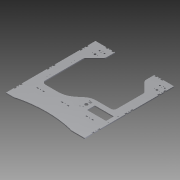
# Autodesk Inventor part: pieza frontal nueva
Saved by Autodesk Inventor 2012 SP1 (Build 160190100, 190)
## iProperties
Created: 2014-12-15
Part Number: pieza frontal nueva
Material: Default
Document SubType Name: Modeling
Designer: PRINCIPAL
Density: 1 g/cm^3
Author: PRINCIPAL
Autodesk Inventor part; units mm, degrees
ref_plane "YZ Plane" through (0, 0, 0) normal (1, 0, 0) x (0, 1, 0)
ref_plane "XZ Plane" through (0, 0, 0) normal (0, 1, 0) x (-1, 0, 0)
ref_plane "XY Plane" through (0, 0, 0) normal (0, 0, 1) x (1, 0, 0)
sketch "Boceto1" plane through (0, 0, 0) normal (0, 0, 1) x (1, 0, 0)
  arc A0 (-182.0823, -56.4965) -> (-184.1823, -54.3965) centre (-184.1823, -56.4965) ccw
  arc A1 (-184.1823, -58.5965) -> (-182.0823, -56.4965) centre (-184.1823, -56.4965) ccw
  arc A2 (-186.2823, -56.4965) -> (-184.1823, -58.5965) centre (-184.1823, -56.4965) ccw
  arc A3 (-184.1823, -54.3965) -> (-186.2823, -56.4965) centre (-184.1823, -56.4965) ccw
  arc A4 (212.9177, -56.4965) -> (210.8177, -54.3965) centre (210.8177, -56.4965) ccw
  arc A5 (210.8177, -58.5965) -> (212.9177, -56.4965) centre (210.8177, -56.4965) ccw
  arc A6 (208.7177, -56.4965) -> (210.8177, -58.5965) centre (210.8177, -56.4965) ccw
  arc A7 (210.8177, -54.3965) -> (208.7177, -56.4965) centre (210.8177, -56.4965) ccw
  arc A8 (206.3177, -154.7797) -> (204.3177, -152.7797) centre (204.3177, -154.7797) ccw
  arc A9 (204.3177, -156.7797) -> (206.3177, -154.7797) centre (204.3177, -154.7797) ccw
  arc A10 (202.3177, -154.7797) -> (204.3177, -156.7797) centre (204.3177, -154.7797) ccw
  arc A11 (204.3177, -152.7797) -> (202.3177, -154.7797) centre (204.3177, -154.7797) ccw
  arc A12 (62.3177, -104.7797) -> (60.3177, -102.7797) centre (60.3177, -104.7797) ccw
  arc A13 (60.3177, -106.7797) -> (62.3177, -104.7797) centre (60.3177, -104.7797) ccw
  arc A14 (58.3177, -104.7797) -> (60.3177, -106.7797) centre (60.3177, -104.7797) ccw
  arc A15 (60.3177, -102.7797) -> (58.3177, -104.7797) centre (60.3177, -104.7797) ccw
  arc A16 (62.3177, -154.7797) -> (60.3177, -152.7797) centre (60.3177, -154.7797) ccw
  arc A17 (60.3177, -156.7797) -> (62.3177, -154.7797) centre (60.3177, -154.7797) ccw
  arc A18 (58.3177, -154.7797) -> (60.3177, -156.7797) centre (60.3177, -154.7797) ccw
  arc A19 (60.3177, -152.7797) -> (58.3177, -154.7797) centre (60.3177, -154.7797) ccw
  arc A20 (206.3177, -104.7797) -> (204.3177, -102.7797) centre (204.3177, -104.7797) ccw
  arc A21 (204.3177, -106.7797) -> (206.3177, -104.7797) centre (204.3177, -104.7797) ccw
  arc A22 (202.3177, -104.7797) -> (204.3177, -106.7797) centre (204.3177, -104.7797) ccw
  arc A23 (204.3177, -102.7797) -> (202.3177, -104.7797) centre (204.3177, -104.7797) ccw
  line L0 (148.3677, -185.9715) -> (158.2677, -185.9715)
  line L1 (158.2677, -185.9715) -> (158.2677, -181.0215)
  line L2 (158.2677, -181.0215) -> (148.3677, -181.0215)
  line L3 (148.3677, -181.0215) -> (148.3677, -185.9715)
  line L4 (33.2677, -185.9715) -> (33.2677, -181.0215)
  line L5 (33.2677, -181.0215) -> (23.3677, -181.0215)
  line L6 (23.3677, -181.0215) -> (23.3677, -185.9715)
  line L7 (23.3677, -185.9715) -> (33.2677, -185.9715)
  line L8 (-91.7323, -185.9715) -> (-91.7323, -181.0215)
  line L9 (-91.7323, -181.0215) -> (-101.6323, -181.0215)
  line L10 (-101.6323, -181.0215) -> (-101.6323, -185.9715)
  line L11 (-101.6323, -185.9715) -> (-91.7323, -185.9715)
  line L12 (3.2677, -185.9715) -> (3.2677, -181.0215)
  line L13 (3.2677, -181.0215) -> (-6.6323, -181.0215)
  line L14 (-6.6323, -181.0215) -> (-6.6323, -185.9715)
  line L15 (-6.6323, -185.9715) -> (3.2677, -185.9715)
  line L16 (-121.7323, -185.9715) -> (-121.7323, -181.0215)
  line L17 (-121.7323, -181.0215) -> (-131.6323, -181.0215)
  line L18 (-131.6323, -181.0215) -> (-131.6323, -185.9715)
  line L19 (-131.6323, -185.9715) -> (-121.7323, -185.9715)
  arc A24 (-109.6823, -183.4965) -> (-111.6823, -181.4965) centre (-111.6823, -183.4965) ccw
  arc A25 (-111.6823, -185.4965) -> (-109.6823, -183.4965) centre (-111.6823, -183.4965) ccw
  arc A26 (-113.6823, -183.4965) -> (-111.6823, -185.4965) centre (-111.6823, -183.4965) ccw
  arc A27 (-111.6823, -181.4965) -> (-113.6823, -183.4965) centre (-111.6823, -183.4965) ccw
  arc A28 (-182.1823, -224.4965) -> (-184.1823, -222.4965) centre (-184.1823, -224.4965) ccw
  arc A29 (-184.1823, -226.4965) -> (-182.1823, -224.4965) centre (-184.1823, -224.4965) ccw
  arc A30 (-186.1823, -224.4965) -> (-184.1823, -226.4965) centre (-184.1823, -224.4965) ccw
  arc A31 (-184.1823, -222.4965) -> (-186.1823, -224.4965) centre (-184.1823, -224.4965) ccw
  arc A32 (15.3177, -183.4965) -> (13.3177, -181.4965) centre (13.3177, -183.4965) ccw
  arc A33 (13.3177, -185.4965) -> (15.3177, -183.4965) centre (13.3177, -183.4965) ccw
  arc A34 (11.3177, -183.4965) -> (13.3177, -185.4965) centre (13.3177, -183.4965) ccw
  arc A35 (13.3177, -181.4965) -> (11.3177, -183.4965) centre (13.3177, -183.4965) ccw
  arc A36 (140.3177, -183.4965) -> (138.3177, -181.4965) centre (138.3177, -183.4965) ccw
  arc A37 (138.3177, -185.4965) -> (140.3177, -183.4965) centre (138.3177, -183.4965) ccw
  arc A38 (136.3177, -183.4965) -> (138.3177, -185.4965) centre (138.3177, -183.4965) ccw
  arc A39 (138.3177, -181.4965) -> (136.3177, -183.4965) centre (138.3177, -183.4965) ccw
  arc A40 (212.8177, -224.4965) -> (210.8177, -222.4965) centre (210.8177, -224.4965) ccw
  arc A41 (210.8177, -226.4965) -> (212.8177, -224.4965) centre (210.8177, -224.4965) ccw
  arc A42 (208.8177, -224.4965) -> (210.8177, -226.4965) centre (210.8177, -224.4965) ccw
  arc A43 (210.8177, -222.4965) -> (208.8177, -224.4965) centre (210.8177, -224.4965) ccw
  line L20 (118.3677, -185.9715) -> (128.2677, -185.9715)
  line L21 (128.2677, -185.9715) -> (128.2677, -181.0215)
  line L22 (128.2677, -181.0215) -> (118.3677, -181.0215)
  line L23 (118.3677, -181.0215) -> (118.3677, -185.9715)
  line L24 (64.9824, -107.508) -> (64.9824, -109.0513)
  line L25 (64.9824, -109.0513) -> (77.3177, -109.0513)
  line L26 (77.3177, -109.0513) -> (77.3177, -107.508)
  line L27 (77.3177, -107.508) -> (64.9824, -107.508)
  line L28 (64.9824, -116.5513) -> (64.9824, -118.0513)
  line L29 (64.9824, -118.0513) -> (77.3177, -118.0513)
  line L30 (77.3177, -118.0513) -> (77.3177, -116.5513)
  line L31 (77.3177, -116.5513) -> (64.9824, -116.5513)
  line L32 (64.9824, -113.5513) -> (64.9824, -115.0513)
  line L33 (64.9824, -115.0513) -> (77.3177, -115.0513)
  line L34 (77.3177, -115.0513) -> (77.3177, -113.5513)
  line L35 (77.3177, -113.5513) -> (64.9824, -113.5513)
  line L36 (77.3177, -112.0513) -> (77.3177, -110.5513)
  line L37 (77.3177, -110.5513) -> (64.9824, -110.5513)
  line L38 (64.9824, -110.5513) -> (64.9824, -112.0513)
  line L39 (64.9824, -112.0513) -> (77.3177, -112.0513)
  arc A44 (72.3677, -148.9787) -> (70.3177, -146.9287) centre (70.3177, -148.9787) ccw
  arc A45 (70.3177, -151.0287) -> (72.3677, -148.9787) centre (70.3177, -148.9787) ccw
  arc A46 (68.2677, -148.9787) -> (70.3177, -151.0287) centre (70.3177, -148.9787) ccw
  arc A47 (70.3177, -146.9287) -> (68.2677, -148.9787) centre (70.3177, -148.9787) ccw
  line L40 (193.1177, -115.2675) -> (193.1177, -154.2918)
  arc A48 (192.8475, -154.5619) -> (193.1177, -154.2918) centre (192.8475, -154.2918) ccw
  line L41 (192.8475, -154.5619) -> (96.7879, -154.5619)
  arc A49 (96.5177, -154.2918) -> (96.7879, -154.5619) centre (96.7879, -154.2918) ccw
  line L42 (96.5177, -154.2918) -> (96.5177, -115.2675)
  arc A50 (96.7879, -114.9974) -> (96.5177, -115.2675) centre (96.7879, -115.2675) ccw
  line L43 (96.7879, -114.9974) -> (192.8475, -114.9974)
  arc A51 (193.1177, -115.2675) -> (192.8475, -114.9974) centre (192.8475, -115.2675) ccw
  arc A52 (62.3177, -132.2797) -> (70.3177, -140.2797) centre (70.3177, -132.2797) ccw
  arc A53 (70.3177, -124.2797) -> (62.3177, -132.2797) centre (70.3177, -132.2797) ccw
  arc A54 (78.3177, -132.2797) -> (70.3177, -124.2797) centre (70.3177, -132.2797) ccw
  arc A55 (70.3177, -140.2797) -> (78.3177, -132.2797) centre (70.3177, -132.2797) ccw
  arc A56 (173.8177, 142.5277) -> (170.3177, 139.0277) centre (173.8177, 139.0277) ccw
  arc A57 (170.3177, 139.0277) -> (173.8177, 135.5277) centre (173.8177, 139.0277) ccw
  arc A58 (173.8177, 135.5277) -> (177.3177, 139.0277) centre (173.8177, 139.0277) ccw
  arc A59 (177.3177, 139.0277) -> (173.8177, 142.5277) centre (173.8177, 139.0277) ccw
  arc A60 (198.8177, 142.5277) -> (195.3177, 139.0277) centre (198.8177, 139.0277) ccw
  arc A61 (195.3177, 139.0277) -> (198.8177, 135.5277) centre (198.8177, 139.0277) ccw
  arc A62 (198.8177, 135.5277) -> (202.3177, 139.0277) centre (198.8177, 139.0277) ccw
  arc A63 (202.3177, 139.0277) -> (198.8177, 142.5277) centre (198.8177, 139.0277) ccw
  arc A64 (186.3177, 135.5777) -> (184.7677, 134.0277) centre (186.3177, 134.0277) ccw
  arc A65 (184.7677, 134.0277) -> (186.3177, 132.4777) centre (186.3177, 134.0277) ccw
  arc A66 (186.3177, 132.4777) -> (187.8677, 134.0277) centre (186.3177, 134.0277) ccw
  arc A67 (187.8677, 134.0277) -> (186.3177, 135.5777) centre (186.3177, 134.0277) ccw
  arc A68 (186.3177, 145.5777) -> (184.7677, 144.0277) centre (186.3177, 144.0277) ccw
  arc A69 (184.7677, 144.0277) -> (186.3177, 142.4777) centre (186.3177, 144.0277) ccw
  arc A70 (186.3177, 142.4777) -> (187.8677, 144.0277) centre (186.3177, 144.0277) ccw
  arc A71 (187.8677, 144.0277) -> (186.3177, 145.5777) centre (186.3177, 144.0277) ccw
  arc A72 (-108.1823, 142.5277) -> (-111.6823, 139.0277) centre (-108.1823, 139.0277) ccw
  arc A73 (-111.6823, 139.0277) -> (-108.1823, 135.5277) centre (-108.1823, 139.0277) ccw
  arc A74 (-108.1823, 135.5277) -> (-104.6823, 139.0277) centre (-108.1823, 139.0277) ccw
  arc A75 (-104.6823, 139.0277) -> (-108.1823, 142.5277) centre (-108.1823, 139.0277) ccw
  arc A76 (-133.1823, 142.5277) -> (-136.6823, 139.0277) centre (-133.1823, 139.0277) ccw
  arc A77 (-136.6823, 139.0277) -> (-133.1823, 135.5277) centre (-133.1823, 139.0277) ccw
  arc A78 (-133.1823, 135.5277) -> (-129.6823, 139.0277) centre (-133.1823, 139.0277) ccw
  arc A79 (-129.6823, 139.0277) -> (-133.1823, 142.5277) centre (-133.1823, 139.0277) ccw
  arc A80 (-120.6823, 135.5777) -> (-122.2323, 134.0277) centre (-120.6823, 134.0277) ccw
  arc A81 (-122.2323, 134.0277) -> (-120.6823, 132.4777) centre (-120.6823, 134.0277) ccw
  arc A82 (-120.6823, 132.4777) -> (-119.1323, 134.0277) centre (-120.6823, 134.0277) ccw
  arc A83 (-119.1323, 134.0277) -> (-120.6823, 135.5777) centre (-120.6823, 134.0277) ccw
  arc A84 (-120.6823, 145.5777) -> (-122.2323, 144.0277) centre (-120.6823, 144.0277) ccw
  arc A85 (-122.2323, 144.0277) -> (-120.6823, 142.4777) centre (-120.6823, 144.0277) ccw
  arc A86 (-120.6823, 142.4777) -> (-119.1323, 144.0277) centre (-120.6823, 144.0277) ccw
  arc A87 (-119.1323, 144.0277) -> (-120.6823, 145.5777) centre (-120.6823, 144.0277) ccw
  arc A88 (173.8177, 113.0777) -> (172.2677, 111.5277) centre (173.8177, 111.5277) ccw
  arc A89 (172.2677, 111.5277) -> (173.8177, 109.9777) centre (173.8177, 111.5277) ccw
  arc A90 (173.8177, 109.9777) -> (175.3677, 111.5277) centre (173.8177, 111.5277) ccw
  arc A91 (175.3677, 111.5277) -> (173.8177, 113.0777) centre (173.8177, 111.5277) ccw
  arc A92 (-116.6823, 113.0777) -> (-118.2323, 111.5277) centre (-116.6823, 111.5277) ccw
  arc A93 (-118.2323, 111.5277) -> (-116.6823, 109.9777) centre (-116.6823, 111.5277) ccw
  arc A94 (-116.6823, 109.9777) -> (-115.1323, 111.5277) centre (-116.6823, 111.5277) ccw
  arc A95 (-115.1323, 111.5277) -> (-116.6823, 113.0777) centre (-116.6823, 111.5277) ccw
  arc A96 (-141.6823, 113.0777) -> (-143.2323, 111.5277) centre (-141.6823, 111.5277) ccw
  arc A97 (-143.2323, 111.5277) -> (-141.6823, 109.9777) centre (-141.6823, 111.5277) ccw
  arc A98 (-141.6823, 109.9777) -> (-140.1323, 111.5277) centre (-141.6823, 111.5277) ccw
  arc A99 (-140.1323, 111.5277) -> (-141.6823, 113.0777) centre (-141.6823, 111.5277) ccw
  arc A100 (198.8177, 113.0777) -> (197.2677, 111.5277) centre (198.8177, 111.5277) ccw
  arc A101 (197.2677, 111.5277) -> (198.8177, 109.9777) centre (198.8177, 111.5277) ccw
  arc A102 (198.8177, 109.9777) -> (200.3677, 111.5277) centre (198.8177, 111.5277) ccw
  arc A103 (200.3677, 111.5277) -> (198.8177, 113.0777) centre (198.8177, 111.5277) ccw
  arc A104 (-111.6823, 171.0277) -> (-113.6823, 169.0277) centre (-111.6823, 169.0277) ccw
  arc A105 (-113.6823, 169.0277) -> (-111.6823, 167.0277) centre (-111.6823, 169.0277) ccw
  arc A106 (-111.6823, 167.0277) -> (-109.6823, 169.0277) centre (-111.6823, 169.0277) ccw
  arc A107 (-109.6823, 169.0277) -> (-111.6823, 171.0277) centre (-111.6823, 169.0277) ccw
  arc A108 (-184.1823, 113.5277) -> (-186.1823, 111.5277) centre (-184.1823, 111.5277) ccw
  arc A109 (-186.1823, 111.5277) -> (-184.1823, 109.5277) centre (-184.1823, 111.5277) ccw
  arc A110 (-184.1823, 109.5277) -> (-182.1823, 111.5277) centre (-184.1823, 111.5277) ccw
  arc A111 (-182.1823, 111.5277) -> (-184.1823, 113.5277) centre (-184.1823, 111.5277) ccw
  arc A112 (210.8177, 113.5277) -> (208.8177, 111.5277) centre (210.8177, 111.5277) ccw
  arc A113 (208.8177, 111.5277) -> (210.8177, 109.5277) centre (210.8177, 111.5277) ccw
  arc A114 (210.8177, 109.5277) -> (212.8177, 111.5277) centre (210.8177, 111.5277) ccw
  arc A115 (212.8177, 111.5277) -> (210.8177, 113.5277) centre (210.8177, 111.5277) ccw
  arc A116 (138.3177, 171.0277) -> (136.3177, 169.0277) centre (138.3177, 169.0277) ccw
  arc A117 (136.3177, 169.0277) -> (138.3177, 167.0277) centre (138.3177, 169.0277) ccw
  arc A118 (138.3177, 167.0277) -> (140.3177, 169.0277) centre (138.3177, 169.0277) ccw
  arc A119 (140.3177, 169.0277) -> (138.3177, 171.0277) centre (138.3177, 169.0277) ccw
  arc A120 (-129.1823, 116.7277) -> (-134.3823, 111.5277) centre (-129.1823, 111.5277) ccw
  arc A121 (-134.3823, 111.5277) -> (-129.1823, 106.3277) centre (-129.1823, 111.5277) ccw
  arc A122 (-129.1823, 106.3277) -> (-123.9823, 111.5277) centre (-129.1823, 111.5277) ccw
  arc A123 (-123.9823, 111.5277) -> (-129.1823, 116.7277) centre (-129.1823, 111.5277) ccw
  arc A124 (186.3177, 116.7277) -> (181.1177, 111.5277) centre (186.3177, 111.5277) ccw
  arc A125 (181.1177, 111.5277) -> (186.3177, 106.3277) centre (186.3177, 111.5277) ccw
  arc A126 (186.3177, 106.3277) -> (191.5177, 111.5277) centre (186.3177, 111.5277) ccw
  arc A127 (191.5177, 111.5277) -> (186.3177, 116.7277) centre (186.3177, 111.5277) ccw
  line L44 (-92.4695, 115.209) -> (-136.2182, 71.4603)
  arc A128 (-136.2182, 71.4603) -> (-140.5823, 60.9244) centre (-125.6823, 60.9244) ccw
  line L45 (-140.5823, 60.9244) -> (-140.5823, -129.0297)
  arc A129 (-140.5823, -129.0297) -> (-120.6823, -148.9297) centre (-120.6823, -129.0297) ccw
  line L46 (-120.6823, -148.9297) -> (-56.306, -148.9297)
  arc A130 (-56.306, -148.9297) -> (0.3907, -131.2823) centre (-56.306, -49.0297) ccw
  arc A131 (0.3907, -131.2823) -> (28.9935, -108.1231) centre (-135.1799, 65.3964) ccw
  arc A132 (77.1714, -88.9436) -> (28.9935, -108.1231) centre (77.1714, -159.0436) ccw
  line L47 (77.1714, -88.9436) -> (152.2606, -88.9436)
  arc A133 (152.2606, -88.9436) -> (167.1606, -74.0436) centre (152.2606, -74.0436) ccw
  line L48 (167.1606, -74.0436) -> (167.1606, 60.9244)
  arc A134 (167.1606, 60.9244) -> (162.7965, 71.4603) centre (152.2606, 60.9244) ccw
  line L49 (162.7965, 71.4603) -> (119.1048, 115.152)
  arc A135 (113.2177, 129.3648) -> (119.1048, 115.152) centre (133.3177, 129.3648) ccw
  line L50 (113.2177, 129.3648) -> (113.2177, 171.6035)
  line L51 (113.2177, 171.6035) -> (118.4177, 171.6035)
  line L52 (118.4177, 171.6035) -> (118.4177, 166.6035)
  line L53 (118.4177, 166.6035) -> (128.2177, 166.6035)
  line L54 (128.2177, 166.6035) -> (128.2177, 171.6035)
  line L55 (128.2177, 171.6035) -> (148.4177, 171.6035)
  line L56 (148.4177, 171.6035) -> (148.4177, 166.6035)
  line L57 (148.4177, 166.6035) -> (158.2177, 166.6035)
  line L58 (158.2177, 166.6035) -> (158.2177, 171.6035)
  line L59 (158.2177, 171.6035) -> (213.4177, 171.6035)
  line L60 (213.4177, 171.6035) -> (213.4177, 131.4035)
  line L61 (213.4177, 131.4035) -> (208.4177, 131.4035)
  line L62 (208.4177, 131.4035) -> (208.4177, 121.6035)
  line L63 (208.4177, 121.6035) -> (213.4177, 121.6035)
  line L64 (213.4177, 121.6035) -> (213.4177, 101.4035)
  line L65 (213.4177, 101.4035) -> (208.4177, 101.4035)
  line L66 (208.4177, 101.4035) -> (208.4177, 91.6035)
  line L67 (208.4177, 91.6035) -> (213.4177, 91.6035)
  line L68 (213.4177, 91.6035) -> (213.4177, -36.5965)
  line L69 (213.4177, -36.5965) -> (208.4177, -36.5965)
  line L70 (208.4177, -36.5965) -> (208.4177, -46.3965)
  line L71 (208.4177, -46.3965) -> (213.4177, -46.3965)
  line L72 (213.4177, -46.3965) -> (213.4177, -66.5965)
  line L73 (213.4177, -66.5965) -> (208.4177, -66.5965)
  line L74 (208.4177, -66.5965) -> (208.4177, -76.3965)
  line L75 (208.4177, -76.3965) -> (213.4177, -76.3965)
  line L76 (213.4177, -76.3965) -> (213.4177, -204.5965)
  line L77 (213.4177, -204.5965) -> (208.4177, -204.5965)
  line L78 (208.4177, -204.5965) -> (208.4177, -214.3965)
  line L79 (208.4177, -214.3965) -> (213.4177, -214.3965)
  line L80 (213.4177, -214.3965) -> (213.4177, -234.5965)
  line L81 (213.4177, -234.5965) -> (208.4177, -234.5965)
  line L82 (208.4177, -234.5965) -> (208.4177, -244.3965)
  line L83 (208.4177, -244.3965) -> (213.4177, -244.3965)
  line L84 (213.4177, -244.3965) -> (213.4177, -284.5965)
  line L85 (213.4177, -284.5965) -> (144.6072, -284.5965)
  line L86 (144.6072, -284.5965) -> (144.5843, -284.5944)
  arc A136 (134.9667, -281.0186) -> (144.5843, -284.5944) centre (1654.6665, 3791.6867) ccw
  arc A137 (134.9667, -281.0186) -> (-134.4811, -281.0186) centre (0.2428, -843.211) ccw
  arc A138 (-144.1217, -284.5965) -> (-134.4811, -281.0186) centre (-232.2812, -32.279) ccw
  line L87 (-144.1217, -284.5965) -> (-186.7823, -284.5965)
  line L88 (-186.7823, -284.5965) -> (-186.7823, -244.3965)
  line L89 (-186.7823, -244.3965) -> (-181.7823, -244.3965)
  line L90 (-181.7823, -244.3965) -> (-181.7823, -234.5965)
  line L91 (-181.7823, -234.5965) -> (-186.7823, -234.5965)
  line L92 (-186.7823, -234.5965) -> (-186.7823, -214.3965)
  line L93 (-186.7823, -214.3965) -> (-181.7823, -214.3965)
  line L94 (-181.7823, -214.3965) -> (-181.7823, -204.5965)
  line L95 (-181.7823, -204.5965) -> (-186.7823, -204.5965)
  line L96 (-186.7823, -204.5965) -> (-186.7823, -76.3965)
  line L97 (-186.7823, -76.3965) -> (-181.7823, -76.3965)
  line L98 (-181.7823, -76.3965) -> (-181.7823, -66.5965)
  line L99 (-181.7823, -66.5965) -> (-186.7823, -66.5965)
  line L100 (-186.7823, -66.5965) -> (-186.7823, -46.3965)
  line L101 (-186.7823, -46.3965) -> (-181.7823, -46.3965)
  line L102 (-181.7823, -46.3965) -> (-181.7823, -36.5965)
  line L103 (-181.7823, -36.5965) -> (-186.7823, -36.5965)
  line L104 (-186.7823, -36.5965) -> (-186.7823, 91.6035)
  line L105 (-186.7823, 91.6035) -> (-181.7823, 91.6035)
  line L106 (-181.7823, 91.6035) -> (-181.7823, 101.4035)
  line L107 (-181.7823, 101.4035) -> (-186.7823, 101.4035)
  line L108 (-186.7823, 101.4035) -> (-186.7823, 121.6035)
  line L109 (-186.7823, 121.6035) -> (-181.7823, 121.6035)
  line L110 (-181.7823, 121.6035) -> (-181.7823, 131.4035)
  line L111 (-181.7823, 131.4035) -> (-186.7823, 131.4035)
  line L112 (-186.7823, 131.4035) -> (-186.7823, 171.6035)
  line L113 (-186.7823, 171.6035) -> (-131.5823, 171.6035)
  line L114 (-131.5823, 171.6035) -> (-131.5823, 166.6035)
  line L115 (-131.5823, 166.6035) -> (-121.7823, 166.6035)
  line L116 (-121.7823, 166.6035) -> (-121.7823, 171.6035)
  line L117 (-121.7823, 171.6035) -> (-101.5823, 171.6035)
  line L118 (-101.5823, 171.6035) -> (-101.5823, 166.6035)
  line L119 (-101.5823, 166.6035) -> (-91.7823, 166.6035)
  line L120 (-91.7823, 166.6035) -> (-91.7823, 171.6035)
  line L121 (-91.7823, 171.6035) -> (-86.5823, 171.6035)
  line L122 (-86.5823, 171.6035) -> (-86.5823, 129.4219)
  arc A139 (-92.4695, 115.209) -> (-86.5823, 129.4219) centre (-106.6823, 129.4219) ccw
  point P0 (0, 0)
  constraints: 280 point on circle, 246 end point, 140 centre point
extrude "Extrusión1" add sketch "Boceto1" along normal blind 5
sketch "Boceto2" plane through (0, 0, 0) normal (0, 0, -1) x (-1, 0, 0)
  line L0 (144.1217, -284.5965) -> (186.7823, -284.5965) projected
  line L1 (186.7823, -204.5965) -> (186.7823, -76.3965) projected
  line L2 (186.7823, -36.5965) -> (186.7823, 91.6035) projected
  circle A0 centre (154.7823, 31.1635) radius 1.25
  circle A1 centre (154.7823, 16.1635) radius 1.25
  circle A2 centre (154.7823, -92.5965) radius 1.25
  circle A3 centre (154.7823, -107.5965) radius 1.25
  point P0 (0, 0)
  dimension "d2" = 2.5
  dimension "d3" = 2.5
  dimension "d4" = 2.5
  dimension "d5" = 2.5
  dimension "d6" = 15
  dimension "d7" = 15
  dimension "d8" = 32
  dimension "d9" = 32
  dimension "d10" = 177
  dimension "d11" = 108.76
  constraints: 4 centre point
  measures "d2" diameter of A0
  measures "d3" diameter of A1
  measures "d4" diameter of A2
  measures "d5" diameter of A3
  measures "d6" distance of A2.centre A3.centre
  measures "d7" distance of A1.centre A0.centre
  measures "d8" distance from line of A1.centre L2
  measures "d9" distance from line of L1 A3.centre
  measures "d10" distance from line of A3.centre L0
  measures "d11" distance of A1.centre A2.centre
extrude "Extrusión2" cut sketch "Boceto2" against normal blind 10
